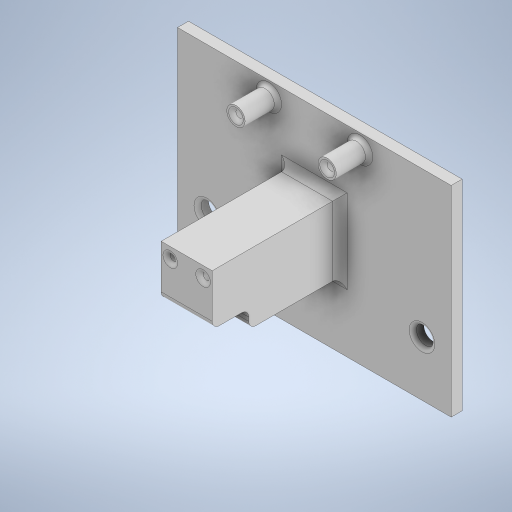
# Autodesk Inventor part: BottomMount
Saved by Autodesk Inventor 2024 (Build 280153000, 153)
## iProperties
Created: 2025-05-17
Part Number: BottomMount
Material: Ogólny
Document SubType Name: Modeling
Designer: Victoria
Density: 1 g/cm^3
Appearance: Domyślna
Author: Victoria
Autodesk Inventor part; units mm, degrees
ref_plane "YZ Plane" through (0, 0, 0) normal (1, 0, 0) x (0, 1, 0)
ref_plane "XZ Plane" through (0, 0, 0) normal (0, 1, 0) x (-1, 0, 0)
ref_plane "XY Plane" through (0, 0, 0) normal (0, 0, 1) x (1, 0, 0)
sketch "Szkic1" plane through (0, 0, 0) normal (0, 0, 1) x (1, 0, 0)
  line L0 (-37.5, -27.5) -> (37.5, -27.5)
  line L1 (37.5, -27.5) -> (37.5, 27.5)
  line L2 (37.5, 27.5) -> (-37.5, 27.5)
  line L3 (-37.5, 27.5) -> (-37.5, -27.5)
  line L4 (-37.5, -27.5) -> (37.5, 27.5) construction
  line L5 (37.5, -27.5) -> (-37.5, 27.5) construction
  circle A0 centre (-29.5, -12.5) radius 2.5
  circle A1 centre (29.5, -12.5) radius 2.5
  point P0 (0, 0)
  dimension "d0" = 75
  dimension "d1" = 55
  dimension "d2" = 5
  dimension "d3" = 5
  constraints: 12 end point, 2 centre point, 2 midpoint, 2 parallel, 1 horizontal, 1 perpendicular
  measures "d0" distance of L2.end L1.end
  measures "d1" distance of L1.end L0.end
  measures "d2" diameter of A0
  measures "d3" diameter of A1
extrude "Wyciągnięcie proste1" add sketch "Szkic1" along normal blind 3
sketch "Szkic2" plane through (0, 0, 3) normal (0, 0, 1) x (1, 0, 0)
  line L0 (-7, 9.5) -> (7, 9.5)
  line L1 (7, 9.5) -> (7, -9.5)
  line L2 (7, -9.5) -> (-7, -9.5)
  line L3 (-7, -9.5) -> (-7, 9.5)
  line L4 (-7, 9.5) -> (7, -9.5) construction
  line L5 (7, 9.5) -> (-7, -9.5) construction
  point P0 (0, 0)
  dimension "d6" = 14
  dimension "d7" = 19
  constraints: 12 end point, 2 midpoint, 2 parallel, 1 horizontal, 1 perpendicular
  measures "d6" distance of L1.end L2.end
  measures "d7" distance of L0.end L1.end
extrude "Wyciągnięcie proste2" add sketch "Szkic2" along normal blind 35
sketch "Szkic3" plane through (0, 0, 38) normal (0, 0, 1) x (1, 0, 0)
  circle A0 centre (-4.5, 6.5) radius 1
  circle A1 centre (4.5, 6.5) radius 1
  line L0 (7, -9.5) -> (-7, -9.5) projected
  line L1 (7, -9.5) -> (7, 9.5) projected
  line L2 (-7, -9.5) -> (7, -9.5)
  line L3 (7, -9.5) -> (7, -4.5)
  line L4 (7, -4.5) -> (-7, -4.5)
  line L5 (-7, -4.5) -> (-7, -9.5)
  point P0 (0, 0)
  dimension "d10" = 2
  dimension "d11" = 2
  dimension "d15" = 5
  constraints: 8 end point, 2 centre point, 2 parallel, 1 horizontal, 1 perpendicular, 1 point on line
  measures "d10" diameter of A0
  measures "d11" diameter of A1
  measures "d15" distance of L3.end L2.end
extrude "Wyciągnięcie proste3" cut sketch "Szkic3" against normal blind 10
fillet "Zaokrąglenie1" radius 2 4 edges at (7, 0, 3) (0, -9.5, 3) (-7, 0, 3) (0, 9.5, 3)
fillet "Zaokrąglenie2" radius 2 3 edges at (0, -4.5, 38) (0, -4.5, 28) (0, -9.5, 28)
sketch "Szkic4" plane through (0, 0, 3) normal (0, 0, 1) x (1, 0, 0)
  line L0 (9, 11.5) -> (-9, 11.5) projected
  circle A0 centre (12.5, 23.5) radius 2.5
  circle A1 centre (-12.5, 23.5) radius 2.5
  circle A2 centre (-12.5, 23.5) radius 1
  circle A3 centre (12.5, 23.5) radius 1
  point P0 (0, 0)
  dimension "d19" = 5
  dimension "d21" = 5
  dimension "d22" = 2
  dimension "d23" = 2
  constraints: 4 centre point, 2 coincident
  measures "d19" diameter of A0
  measures "d21" diameter of A1
  measures "d22" diameter of A2
  measures "d23" diameter of A3
extrude "Wyciągnięcie proste4" add sketch "Szkic4" along normal blind 9
fillet "Zaokrąglenie3" radius 1 8 edges at (-15, 23.5, 3) (10, 23.5, 3) (11.5, 23.5, 12) (-13.5, 23.5, 12) (-5.5, 6.5, 38) (3.5, 6.5, 38) (-32, -12.5, 3) (27, -12.5, 3)
